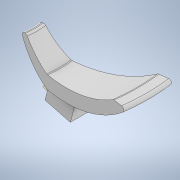
# Autodesk Inventor part: 8003_base_250uH_DCore_2layer_Tx_Filter_MPSv2_v1
Saved by Autodesk Inventor 2021 (Build 250183000, 183)
## iProperties
Created: 2021-02-24
Part Number: 8003_base_250uH_DCore_2layer_Tx_Filter_MPSv2_v1
Material: Generic
Document SubType Name: Modeling
Designer: Barksdale
Density: 1 g/cm^3
Appearance: Default
Author: Barksdale
Autodesk Inventor part; units mm, degrees
ref_plane "YZ Plane" through (0, 0, 0) normal (1, 0, 0) x (0, 1, 0)
ref_plane "XZ Plane" through (0, 0, 0) normal (0, 1, 0) x (-1, 0, 0)
ref_plane "XY Plane" through (0, 0, 0) normal (0, 0, 1) x (1, 0, 0)
sketch "Sketch1" plane through (0, 0, 0) normal (0, 0, 1) x (1, 0, 0)
  arc A0 (13.5052, -15.3166) -> (17.8054, -19.1492) centre (23.1488, -8.825) ccw
  line L0 (17.9048, -19.2) -> (17.9048, -21.7)
  arc A1 (12.4145, -15.7877) -> (17.8054, -21.6492) centre (23.1488, -11.325) ccw
  arc A2 (18.015, -21.7047) -> (34.7578, -15.9783) centre (19.0075, 2.7328) ccw
  arc A3 (18.015, -19.2047) -> (32.4817, -15.1785) centre (19.0075, 5.2328) ccw
  arc A4 (43.4332, 3.9828) -> (43.4613, 4.8) centre (19.0075, 5.2328) ccw
  line L1 (12.8762, -15.0958) -> (13.0904, -15.0958)
  line L2 (32.7572, -15.0958) -> (34.4358, -15.0958)
  arc A5 (13.5052, -15.3166) -> (13.0904, -15.0958) centre (13.0904, -15.5958) ccw
  arc A6 (12.8762, -15.0958) -> (12.4145, -15.7877) centre (12.8762, -15.5958) ccw
  arc A7 (32.7572, -15.0958) -> (32.4817, -15.1785) centre (32.7572, -15.5958) ccw
  arc A8 (34.7578, -15.9783) -> (34.4358, -15.0958) centre (34.4358, -15.5958) ccw
  arc A9 (17.8054, -21.6492) -> (18.015, -21.7047) centre (18.0352, -21.2051) ccw
  arc A10 (17.8054, -19.1492) -> (18.015, -19.2047) centre (18.0352, -18.7051) ccw
  line L3 (0, 0) -> (0, -27.4347)
  point P0 (13.3602, -15.0958)
  point P1 (12.1524, -15.0958)
  point P2 (35.7502, -15.0958)
  point P3 (32.6062, -15.0958)
  dimension "d0" = 2.5
  dimension "d1" = 0.5
  constraints: 29 point on circle, 12 tangent, 11 centre point, 8 end point, 5 equal radius, 4 point on line, 2 vertical
  measures "d0" distance of L0.start L0.end
  measures "d1" radius of A5
revolve "Revolution1" add sketch "Sketch1" angle 7.5 about axis through (0, 0, 0) along (0, -1, 0) and the other way 7.5
ref_plane "Work Plane1" through (17.6531, -21.6492, 2.3241) normal (0.258269, 0.966073, 0) x (0.9583529, -0.2562051, 0.1261695)
sketch "Sketch2" plane through (17.6531, -21.6492, 2.3241) normal (0.258269, 0.966073, 0) x (0.9583529, -0.2562051, 0.1261695)
  line L0 (0.2147, -0.0004) -> (-0.3768, 4.6654)
  line L1 (0.2147, -0.0004) -> (5.1719, 0.6523)
  line L2 (0.2147, -0.0004) -> (5.2147, -0.0004) construction
  line L3 (5.1719, 0.6523) -> (4.5581, 5.3151)
  line L4 (4.5581, 5.3151) -> (-0.3768, 4.6654)
  point P0 (-22.7578, -0.5517)
  dimension "d4" = 4.6658
  dimension "d5" = 5
  dimension "d6" = 7.5
  constraints: 10 end point, 2 perpendicular, 1 equal length, 1 horizontal
  measures "d4" vertical distance of L0.start L0.end
  measures "d5" distance of L0.start L1.end
  measures "d6" angle of L2 L1
extrude "Extrusion1" add sketch "Sketch2" along normal blind 2 and the other way blind 2
body "Solid1"
